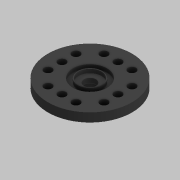
# Autodesk Inventor part: MG서보모터 원형부품
Saved by Autodesk Inventor 2021 (Build 250183000, 183)
## iProperties
Created: 2021-09-03
Part Number: MG서보모터 원형부품
Material: 일반
Document SubType Name: Modeling
Designer: fly01
Density: 1 g/cm^3
Appearance: 기본값
Author: fly01
Autodesk Inventor part; units mm, degrees
ref_plane "YZ Plane" through (0, 0, 0) normal (1, 0, 0) x (0, 1, 0)
ref_plane "XZ Plane" through (0, 0, 0) normal (0, 1, 0) x (-1, 0, 0)
ref_plane "XY Plane" through (0, 0, 0) normal (0, 0, 1) x (1, 0, 0)
sketch "스케치1" plane through (0, 0, 0) normal (0, 1, 0) x (-1, 0, 0)
  circle A0 centre (0, 0) radius 4.35
  circle A1 centre (0, 0) radius 2.75
  dimension "d0" = 8.7
  dimension "d1" = 5.5
  constraints: 2 centre point, 2 coincident
  measures "d0" diameter of A0
  measures "d1" diameter of A1
extrude "돌출1" add sketch "스케치1" against normal blind 3
sketch "스케치3" plane through (0, 0, 0) normal (0, 1, 0) x (1, 0, 0)
  circle A0 centre (0, 0) radius 10.5
  circle A1 centre (0, 0) radius 1.5
  dimension "d4" = 21
  dimension "d5" = 3
  constraints: 2 centre point, 2 coincident
  measures "d4" diameter of A0
  measures "d5" diameter of A1
extrude "돌출2" add sketch "스케치3" along normal blind 2.2
sketch "스케치4" plane through (0, 2.2, 0) normal (0, 1, 0) x (1, 0, 0)
  circle A0 centre (0, 0) radius 2.85
  circle A1 centre (0, 0) radius 3.05
  circle A2 centre (0, 0) radius 4.25
  dimension "d8" = 5.7
  dimension "d9" = 6.1
  dimension "d10" = 8.5
  constraints: 3 centre point, 3 coincident
  measures "d8" diameter of A0
  measures "d9" diameter of A1
  measures "d10" diameter of A2
extrude "돌출3" cut sketch "스케치4" against normal blind 1
sketch "스케치5" plane through (0, 2.2, 0) normal (0, 1, 0) x (1, 0, 0)
  circle A0 centre (-7, 0) radius 1
  circle A1 centre (-7, -3.5) radius 1
  line L0 (0, 0) -> (-0.944, 0)
  circle A2 centre (-7, 3.5) radius 1
  dimension "d13" = 2
  dimension "d14" = 7
  dimension "d15" = 2
  dimension "d16" = 3.5
  constraints: 3 centre point, 2 end point, 1 horizontal, 1 symmetric about line, 1 other
  measures "d13" diameter of A0
  measures "d14" distance of L0.start A0.centre
  measures "d15" diameter of A1
  measures "d16" distance of A0.centre A1.centre
extrude "돌출4" cut sketch "스케치5" against normal blind 7.25
pattern_circular "원형 패턴1" count 4 over 360 about axis through (0, 2.2, 0) along (0, -1, 0) of "돌출4"
